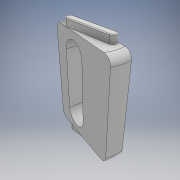
# Autodesk Inventor part: 相机锁台
Saved by Autodesk Inventor 2018.2 (Build 222227000, 227)
## iProperties
Created: 2017-12-28
Part Number: 相机锁台
Material: 常规
Document SubType Name: Modeling
Designer: Administrator
Density: 1 g/cm^3
Appearance: 默认
Author: Administrator
Autodesk Inventor part; units mm, degrees
ref_plane "YZ Plane" through (0, 0, 0) normal (1, 0, 0) x (0, 1, 0)
ref_plane "XZ Plane" through (0, 0, 0) normal (0, 1, 0) x (-1, 0, 0)
sketch "草图1" plane through (0, 0, 0) normal (0, 0, 1) x (1, 0, 0)
  line L0 (-9, 0) -> (9, 0)
  line L1 (-7, 0) -> (7, 0)
  arc A0 (-9.7, 4.6509) -> (-10.7572, 0.072) centre (0, 0) ccw
  arc A1 (9.7, -4.6509) -> (10.7572, -0.072) centre (0, 0) ccw
  line L2 (7, 0) -> (-3, 0)
  line L3 (-6.5, 0) -> (0.5, 0)
  line L4 (-6.5, 0) -> (-5.6425, 3.7142)
  line L5 (-6.5, 0) -> (-6.6996, -0.8648)
  line L6 (0.5, 0) -> (1.0033, 2.1799)
  line L7 (0.5, 0) -> (-0.0539, -2.3991)
  line L8 (-7, 0) -> (7, 0) construction
  line L9 (-6, -1) -> (6, -1)
  line L10 (6, 1) -> (-6, 1)
  arc A2 (-6, 1) -> (-6, -1) centre (-6, 0) ccw
  arc A3 (6, -1) -> (6, 1) centre (6, 0) ccw
  line L11 (-10.7572, 0.072) -> (-6.6996, -0.8648)
  line L12 (-9.7, 4.6509) -> (10.7572, -0.072)
  line L13 (-6.6996, -0.8648) -> (-0.0539, -2.3991)
  line L14 (-0.0539, -2.3991) -> (9.7, -4.6509)
  point P0 (0, 0)
  dimension "d0" = 18
  dimension "d1" = 14
  dimension "d3" = 10
  dimension "d4" = 7
  dimension "d9" = 2
  constraints: 32 end point, 11 point on circle, 8 point on line, 8 tangent, 6 coincident, 4 centre point, 4 midpoint, 4 parallel, 4 perpendicular, 3 horizontal, 1 collinear
  measures "d0" distance of L0.start L0.end
  measures "d1" distance of L1.end L1.start
  measures "d3" distance of L1.end L2.end
  measures "d4" distance of L3.end L3.start
  measures "d9" diameter of A3
ref_plane "工作平面1" through (-6.6996, -0.8648, 0) normal (0.2249511, 0.9743701, 0) x (-0.9743701, 0.2249511, 0)
sketch "草图3" plane through (-6.6996, -0.8648, 0) normal (0.2249511, 0.9743701, 0) x (-0.9743701, 0.2249511, 0)
  line L0 (4.1642, 0) -> (-16.8311, 0) projected
  line L1 (0, 0) -> (-6.8206, 0) projected
  line L2 (-3.4103, 8.5) -> (-3.4103, -8.5) construction
  line L3 (-6.9103, 8.5) -> (-6.9103, -8.5)
  line L4 (0.0897, -8.5) -> (0.0897, 8.5)
  arc A0 (0.0897, 8.5) -> (-6.9103, 8.5) centre (-3.4103, 8.5) ccw
  arc A1 (-6.9103, -8.5) -> (0.0897, -8.5) centre (-3.4103, -8.5) ccw
  point P0 (-6.3334, 0)
  point P1 (-3.4103, 0)
  point P2 (-3.4103, 0)
  dimension "d10" = 8.5
  dimension "d11" = 7
  constraints: 8 end point, 5 coincident, 4 point on circle, 4 tangent, 2 centre point, 2 midpoint, 1 parallel, 1 vertical
  measures "d10" distance of point (-3.41, 0) L2.end
  measures "d11" diameter of A1
extrude "拉伸1" add sketch "草图1" along normal mid plane 28
ref_plane "工作平面2" through (0, 0, 0) normal (0, 0, 1) x (1, 0, 0)
sketch "草图4" plane through (0, 0, 0) normal (0, 0, 1) x (1, 0, 0)
  arc A0 (6, -1) -> (6, 1) centre (6, 0) ccw projected
  line L0 (6, 1) -> (-6, 1) projected
  arc A1 (-6, 1) -> (-6, -1) centre (-6, 0) ccw projected
  line L1 (-6, -1) -> (6, -1) projected
  point P0 (0, 0)
extrude "拉伸2" add sketch "草图4" along normal mid plane 32
extrude "拉伸3" cut sketch "草图3" along normal blind 32
fillet "圆角1" radius 0.139 1 edges at (0, 1, -16)
fillet "圆角2" radius 0.213 1 edges at (0, 1, 16)
fillet "圆角3" radius 2 4 edges at (-10.4817, 2.4199, 14) (-10.4817, 2.4199, -14) (10.4817, -2.4199, 14) (10.4817, -2.4199, -14)
